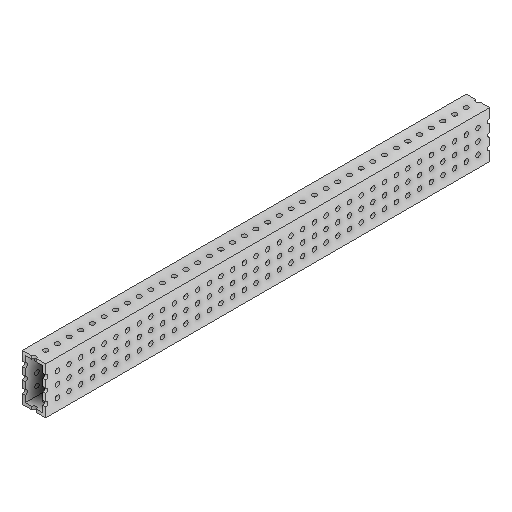
# Autodesk Inventor part: Forja - Base Chassi
Saved by Autodesk Inventor 2027.1 (Build 311270010, 270A)
## iProperties
Created: 2026-05-13
Part Number: Forja - Base Chassi
Material: Genérico
Document SubType Name: Modeling
Designer: djair.oliveira
Density: 1 g/cm^3
Appearance: Padrão
Author: djair.oliveira
Autodesk Inventor part; units mm, degrees
ref_plane "YZ Plane" through (0, 0, 0) normal (1, 0, 0) x (0, 1, 0)
ref_plane "XZ Plane" through (0, 0, 0) normal (0, 1, 0) x (-1, 0, 0)
ref_plane "XY Plane" through (0, 0, 0) normal (0, 0, 1) x (1, 0, 0)
sketch "Esboço1" plane through (0, 0, 0) normal (0, 0, 1) x (1, 0, 0)
  line L0 (12.7, -25.4) -> (-12.7, -25.4)
  line L1 (-12.7, -25.4) -> (-12.7, 25.4)
  line L2 (-12.7, 25.4) -> (12.7, 25.4)
  line L3 (12.7, 25.4) -> (12.7, -25.4)
  line L4 (12.7, -25.4) -> (-12.7, 25.4) construction
  line L5 (-12.7, -25.4) -> (12.7, 25.4) construction
  line L6 (9.525, -22.225) -> (-9.525, -22.225)
  line L7 (-9.525, -22.225) -> (-9.525, 22.225)
  line L8 (-9.525, 22.225) -> (9.525, 22.225)
  line L9 (9.525, 22.225) -> (9.525, -22.225)
  line L10 (9.525, -22.225) -> (-9.525, 22.225) construction
  line L11 (-9.525, -22.225) -> (9.525, 22.225) construction
  point P0 (0, 0)
  dimension "d1" = 3.175
  dimension "d2" = 3.175
  dimension "d3" = 25.4
  dimension "d4" = 50.8
  constraints: 24 end point, 4 midpoint, 4 parallel, 2 horizontal, 2 perpendicular
  measures "d1" distance between parallel lines of L1 L7
  measures "d2" distance between parallel lines of L2 L8
  measures "d3" distance of L1.end L2.end
  measures "d4" distance of L2.end L0.start
extrude "Extrusão1" add sketch "Esboço1" along normal blind 482.6
sketch "Esboço2" plane through (-12.7, 25.4, 0) normal (0, 1, 0) x (1, 0, 0)
  circle A0 centre (12.7, -241.3) radius 2.5
  line L0 (0, 0) -> (0, -482.6) projected
  line L1 (25.4, -482.6) -> (0, -482.6) projected
  line L2 (25.4, 0) -> (0, 0) projected
  circle A1 centre (12.7, -254) radius 2.5
  circle A2 centre (12.7, -228.6) radius 2.5
  circle A3 centre (12.7, -266.7) radius 2.5
  circle A4 centre (12.7, -215.9) radius 2.5
  circle A5 centre (12.7, -279.4) radius 2.5
  circle A6 centre (12.7, -203.2) radius 2.5
  circle A7 centre (12.7, -292.1) radius 2.5
  circle A8 centre (12.7, -190.5) radius 2.5
  circle A9 centre (12.7, -304.8) radius 2.5
  circle A10 centre (12.7, -177.8) radius 2.5
  circle A11 centre (12.7, -317.5) radius 2.5
  circle A12 centre (12.7, -165.1) radius 2.5
  circle A13 centre (12.7, -330.2) radius 2.5
  circle A14 centre (12.7, -152.4) radius 2.5
  circle A15 centre (12.7, -342.9) radius 2.5
  circle A16 centre (12.7, -139.7) radius 2.5
  circle A17 centre (12.7, -355.6) radius 2.5
  circle A18 centre (12.7, -127) radius 2.5
  circle A19 centre (12.7, -368.3) radius 2.5
  circle A20 centre (12.7, -114.3) radius 2.5
  circle A21 centre (12.7, -381) radius 2.5
  circle A22 centre (12.7, -101.6) radius 2.5
  circle A23 centre (12.7, -393.7) radius 2.5
  circle A24 centre (12.7, -88.9) radius 2.5
  circle A25 centre (12.7, -406.4) radius 2.5
  circle A26 centre (12.7, -76.2) radius 2.5
  circle A27 centre (12.7, -419.1) radius 2.5
  circle A28 centre (12.7, -63.5) radius 2.5
  circle A29 centre (12.7, -431.8) radius 2.5
  circle A30 centre (12.7, -50.8) radius 2.5
  circle A31 centre (12.7, -444.5) radius 2.5
  circle A32 centre (12.7, -38.1) radius 2.5
  circle A33 centre (12.7, -457.2) radius 2.5
  circle A34 centre (12.7, -25.4) radius 2.5
  circle A35 centre (12.7, -469.9) radius 2.5
  circle A36 centre (12.7, -12.7) radius 2.5
  circle A37 centre (12.7, -482.6) radius 2.5
  circle A38 centre (12.7, 0) radius 2.5
  circle A39 centre (12.7, -495.3) radius 2.5
  circle A40 centre (12.7, 12.7) radius 2.5
  circle A41 centre (12.7, -508) radius 2.5
  circle A42 centre (12.7, 25.4) radius 2.5
  circle A43 centre (12.7, -520.7) radius 2.5
  circle A44 centre (12.7, 38.1) radius 2.5
  circle A45 centre (12.7, -533.4) radius 2.5
  circle A46 centre (12.7, 50.8) radius 2.5
  circle A47 centre (12.7, -546.1) radius 2.5
  circle A48 centre (12.7, 63.5) radius 2.5
  circle A49 centre (12.7, -558.8) radius 2.5
  circle A50 centre (12.7, 76.2) radius 2.5
  circle A51 centre (12.7, -571.5) radius 2.5
  circle A52 centre (12.7, 88.9) radius 2.5
  circle A53 centre (12.7, -584.2) radius 2.5
  circle A54 centre (12.7, 101.6) radius 2.5
  circle A55 centre (12.7, -596.9) radius 2.5
  circle A56 centre (12.7, 114.3) radius 2.5
  circle A57 centre (12.7, -609.6) radius 2.5
  circle A58 centre (12.7, 127) radius 2.5
  circle A59 centre (12.7, -622.3) radius 2.5
  circle A60 centre (12.7, 139.7) radius 2.5
  circle A61 centre (12.7, -635) radius 2.5
  circle A62 centre (12.7, 152.4) radius 2.5
  circle A63 centre (12.7, -647.7) radius 2.5
  circle A64 centre (12.7, 165.1) radius 2.5
  circle A65 centre (12.7, -660.4) radius 2.5
  circle A66 centre (12.7, 177.8) radius 2.5
  circle A67 centre (12.7, -673.1) radius 2.5
  circle A68 centre (12.7, 190.5) radius 2.5
  circle A69 centre (12.7, -685.8) radius 2.5
  circle A70 centre (12.7, 203.2) radius 2.5
  point P0 (12.7, 0)
  point P1 (12.7, -482.6)
  point P2 (12.7, 0)
  point P3 (12.7, 0)
  dimension "d7" = 5
  dimension "d8" = 12.7
  dimension "d9" = 482.6
  dimension "d10" = 241.3
  dimension "d13" = 12.7
  constraints: 71 centre point, 3 midpoint, 1 vertical, 140 other
  measures "d7" diameter of A0
  measures "d8" distance from line of L0 A0.centre
  measures "d9" distance of point (12.7, -482.6) point (12.7, 0)
  measures "d10" distance of point (12.7, 0) A0.centre
  measures "d13" distance of A0.centre A1.centre
extrude "Extrusão2" cut sketch "Esboço2" against normal up to surface (50.8 mm away)
sketch "Esboço3" plane through (12.7, -25.4, 0) normal (1, 0, 0) x (0, 0, -1)
  circle A0 centre (-241.3, 38.1) radius 2.5
  circle A1 centre (-241.3, 25.4) radius 2.5
  circle A2 centre (-241.3, 12.7) radius 2.5
  line L0 (0, 50.8) -> (-482.6, 50.8) projected
  line L1 (-241.3, 50.8) -> (-241.3, 0)
  line L2 (0, 0) -> (-482.6, 0) projected
  circle A3 centre (-254, 38.1) radius 2.5
  circle A4 centre (-254, 25.4) radius 2.5
  circle A5 centre (-254, 12.7) radius 2.5
  circle A6 centre (-228.6, 38.1) radius 2.5
  circle A7 centre (-228.6, 25.4) radius 2.5
  circle A8 centre (-228.6, 12.7) radius 2.5
  circle A9 centre (-266.7, 38.1) radius 2.5
  circle A10 centre (-266.7, 25.4) radius 2.5
  circle A11 centre (-266.7, 12.7) radius 2.5
  circle A12 centre (-215.9, 38.1) radius 2.5
  circle A13 centre (-215.9, 25.4) radius 2.5
  circle A14 centre (-215.9, 12.7) radius 2.5
  circle A15 centre (-279.4, 38.1) radius 2.5
  circle A16 centre (-279.4, 25.4) radius 2.5
  circle A17 centre (-279.4, 12.7) radius 2.5
  circle A18 centre (-203.2, 38.1) radius 2.5
  circle A19 centre (-203.2, 25.4) radius 2.5
  circle A20 centre (-203.2, 12.7) radius 2.5
  circle A21 centre (-292.1, 38.1) radius 2.5
  circle A22 centre (-292.1, 25.4) radius 2.5
  circle A23 centre (-292.1, 12.7) radius 2.5
  circle A24 centre (-190.5, 38.1) radius 2.5
  circle A25 centre (-190.5, 25.4) radius 2.5
  circle A26 centre (-190.5, 12.7) radius 2.5
  circle A27 centre (-304.8, 38.1) radius 2.5
  circle A28 centre (-304.8, 25.4) radius 2.5
  circle A29 centre (-304.8, 12.7) radius 2.5
  circle A30 centre (-177.8, 38.1) radius 2.5
  circle A31 centre (-177.8, 25.4) radius 2.5
  circle A32 centre (-177.8, 12.7) radius 2.5
  circle A33 centre (-317.5, 38.1) radius 2.5
  circle A34 centre (-317.5, 25.4) radius 2.5
  circle A35 centre (-317.5, 12.7) radius 2.5
  circle A36 centre (-165.1, 38.1) radius 2.5
  circle A37 centre (-165.1, 25.4) radius 2.5
  circle A38 centre (-165.1, 12.7) radius 2.5
  circle A39 centre (-330.2, 38.1) radius 2.5
  circle A40 centre (-330.2, 25.4) radius 2.5
  circle A41 centre (-330.2, 12.7) radius 2.5
  circle A42 centre (-152.4, 38.1) radius 2.5
  circle A43 centre (-152.4, 25.4) radius 2.5
  circle A44 centre (-152.4, 12.7) radius 2.5
  circle A45 centre (-342.9, 38.1) radius 2.5
  circle A46 centre (-342.9, 25.4) radius 2.5
  circle A47 centre (-342.9, 12.7) radius 2.5
  circle A48 centre (-139.7, 38.1) radius 2.5
  circle A49 centre (-139.7, 25.4) radius 2.5
  circle A50 centre (-139.7, 12.7) radius 2.5
  circle A51 centre (-355.6, 38.1) radius 2.5
  circle A52 centre (-355.6, 25.4) radius 2.5
  circle A53 centre (-355.6, 12.7) radius 2.5
  circle A54 centre (-127, 38.1) radius 2.5
  circle A55 centre (-127, 25.4) radius 2.5
  circle A56 centre (-127, 12.7) radius 2.5
  circle A57 centre (-368.3, 38.1) radius 2.5
  circle A58 centre (-368.3, 25.4) radius 2.5
  circle A59 centre (-368.3, 12.7) radius 2.5
  circle A60 centre (-114.3, 38.1) radius 2.5
  circle A61 centre (-114.3, 25.4) radius 2.5
  circle A62 centre (-114.3, 12.7) radius 2.5
  circle A63 centre (-381, 38.1) radius 2.5
  circle A64 centre (-381, 25.4) radius 2.5
  circle A65 centre (-381, 12.7) radius 2.5
  circle A66 centre (-101.6, 38.1) radius 2.5
  circle A67 centre (-101.6, 25.4) radius 2.5
  circle A68 centre (-101.6, 12.7) radius 2.5
  circle A69 centre (-393.7, 38.1) radius 2.5
  circle A70 centre (-393.7, 25.4) radius 2.5
  circle A71 centre (-393.7, 12.7) radius 2.5
  circle A72 centre (-88.9, 38.1) radius 2.5
  circle A73 centre (-88.9, 25.4) radius 2.5
  circle A74 centre (-88.9, 12.7) radius 2.5
  circle A75 centre (-406.4, 38.1) radius 2.5
  circle A76 centre (-406.4, 25.4) radius 2.5
  circle A77 centre (-406.4, 12.7) radius 2.5
  circle A78 centre (-76.2, 38.1) radius 2.5
  circle A79 centre (-76.2, 25.4) radius 2.5
  circle A80 centre (-76.2, 12.7) radius 2.5
  circle A81 centre (-419.1, 38.1) radius 2.5
  circle A82 centre (-419.1, 25.4) radius 2.5
  circle A83 centre (-419.1, 12.7) radius 2.5
  circle A84 centre (-63.5, 38.1) radius 2.5
  circle A85 centre (-63.5, 25.4) radius 2.5
  circle A86 centre (-63.5, 12.7) radius 2.5
  circle A87 centre (-431.8, 38.1) radius 2.5
  circle A88 centre (-431.8, 25.4) radius 2.5
  circle A89 centre (-431.8, 12.7) radius 2.5
  circle A90 centre (-50.8, 38.1) radius 2.5
  circle A91 centre (-50.8, 25.4) radius 2.5
  circle A92 centre (-50.8, 12.7) radius 2.5
  circle A93 centre (-444.5, 38.1) radius 2.5
  circle A94 centre (-444.5, 25.4) radius 2.5
  circle A95 centre (-444.5, 12.7) radius 2.5
  circle A96 centre (-38.1, 38.1) radius 2.5
  circle A97 centre (-38.1, 25.4) radius 2.5
  circle A98 centre (-38.1, 12.7) radius 2.5
  circle A99 centre (-457.2, 38.1) radius 2.5
  circle A100 centre (-457.2, 25.4) radius 2.5
  circle A101 centre (-457.2, 12.7) radius 2.5
  circle A102 centre (-25.4, 38.1) radius 2.5
  circle A103 centre (-25.4, 25.4) radius 2.5
  circle A104 centre (-25.4, 12.7) radius 2.5
  circle A105 centre (-469.9, 38.1) radius 2.5
  circle A106 centre (-469.9, 25.4) radius 2.5
  circle A107 centre (-469.9, 12.7) radius 2.5
  circle A108 centre (-12.7, 38.1) radius 2.5
  circle A109 centre (-12.7, 25.4) radius 2.5
  circle A110 centre (-12.7, 12.7) radius 2.5
  circle A111 centre (-482.6, 38.1) radius 2.5
  circle A112 centre (-482.6, 25.4) radius 2.5
  circle A113 centre (-482.6, 12.7) radius 2.5
  circle A114 centre (0, 38.1) radius 2.5
  circle A115 centre (0, 25.4) radius 2.5
  circle A116 centre (0, 12.7) radius 2.5
  circle A117 centre (-495.3, 38.1) radius 2.5
  circle A118 centre (-495.3, 25.4) radius 2.5
  circle A119 centre (-495.3, 12.7) radius 2.5
  circle A120 centre (12.7, 38.1) radius 2.5
  circle A121 centre (12.7, 25.4) radius 2.5
  circle A122 centre (12.7, 12.7) radius 2.5
  circle A123 centre (-508, 38.1) radius 2.5
  circle A124 centre (-508, 25.4) radius 2.5
  circle A125 centre (-508, 12.7) radius 2.5
  circle A126 centre (25.4, 38.1) radius 2.5
  circle A127 centre (25.4, 25.4) radius 2.5
  circle A128 centre (25.4, 12.7) radius 2.5
  circle A129 centre (-520.7, 38.1) radius 2.5
  circle A130 centre (-520.7, 25.4) radius 2.5
  circle A131 centre (-520.7, 12.7) radius 2.5
  circle A132 centre (38.1, 38.1) radius 2.5
  circle A133 centre (38.1, 25.4) radius 2.5
  circle A134 centre (38.1, 12.7) radius 2.5
  circle A135 centre (-533.4, 38.1) radius 2.5
  circle A136 centre (-533.4, 25.4) radius 2.5
  circle A137 centre (-533.4, 12.7) radius 2.5
  circle A138 centre (50.8, 38.1) radius 2.5
  circle A139 centre (50.8, 25.4) radius 2.5
  circle A140 centre (50.8, 12.7) radius 2.5
  circle A141 centre (-546.1, 38.1) radius 2.5
  circle A142 centre (-546.1, 25.4) radius 2.5
  circle A143 centre (-546.1, 12.7) radius 2.5
  circle A144 centre (63.5, 38.1) radius 2.5
  circle A145 centre (63.5, 25.4) radius 2.5
  circle A146 centre (63.5, 12.7) radius 2.5
  circle A147 centre (-558.8, 38.1) radius 2.5
  circle A148 centre (-558.8, 25.4) radius 2.5
  circle A149 centre (-558.8, 12.7) radius 2.5
  circle A150 centre (76.2, 38.1) radius 2.5
  circle A151 centre (76.2, 25.4) radius 2.5
  circle A152 centre (76.2, 12.7) radius 2.5
  circle A153 centre (-571.5, 38.1) radius 2.5
  circle A154 centre (-571.5, 25.4) radius 2.5
  circle A155 centre (-571.5, 12.7) radius 2.5
  circle A156 centre (88.9, 38.1) radius 2.5
  circle A157 centre (88.9, 25.4) radius 2.5
  circle A158 centre (88.9, 12.7) radius 2.5
  circle A159 centre (-584.2, 38.1) radius 2.5
  circle A160 centre (-584.2, 25.4) radius 2.5
  circle A161 centre (-584.2, 12.7) radius 2.5
  circle A162 centre (101.6, 38.1) radius 2.5
  circle A163 centre (101.6, 25.4) radius 2.5
  circle A164 centre (101.6, 12.7) radius 2.5
  circle A165 centre (-596.9, 38.1) radius 2.5
  circle A166 centre (-596.9, 25.4) radius 2.5
  circle A167 centre (-596.9, 12.7) radius 2.5
  circle A168 centre (114.3, 38.1) radius 2.5
  circle A169 centre (114.3, 25.4) radius 2.5
  circle A170 centre (114.3, 12.7) radius 2.5
  circle A171 centre (-609.6, 38.1) radius 2.5
  circle A172 centre (-609.6, 25.4) radius 2.5
  circle A173 centre (-609.6, 12.7) radius 2.5
  circle A174 centre (127, 38.1) radius 2.5
  circle A175 centre (127, 25.4) radius 2.5
  circle A176 centre (127, 12.7) radius 2.5
  circle A177 centre (-622.3, 38.1) radius 2.5
  circle A178 centre (-622.3, 25.4) radius 2.5
  circle A179 centre (-622.3, 12.7) radius 2.5
  circle A180 centre (139.7, 38.1) radius 2.5
  circle A181 centre (139.7, 25.4) radius 2.5
  circle A182 centre (139.7, 12.7) radius 2.5
  circle A183 centre (-635, 38.1) radius 2.5
  circle A184 centre (-635, 25.4) radius 2.5
  circle A185 centre (-635, 12.7) radius 2.5
  circle A186 centre (152.4, 38.1) radius 2.5
  circle A187 centre (152.4, 25.4) radius 2.5
  circle A188 centre (152.4, 12.7) radius 2.5
  circle A189 centre (-647.7, 38.1) radius 2.5
  circle A190 centre (-647.7, 25.4) radius 2.5
  circle A191 centre (-647.7, 12.7) radius 2.5
  circle A192 centre (165.1, 38.1) radius 2.5
  circle A193 centre (165.1, 25.4) radius 2.5
  circle A194 centre (165.1, 12.7) radius 2.5
  circle A195 centre (-660.4, 38.1) radius 2.5
  circle A196 centre (-660.4, 25.4) radius 2.5
  circle A197 centre (-660.4, 12.7) radius 2.5
  circle A198 centre (177.8, 38.1) radius 2.5
  circle A199 centre (177.8, 25.4) radius 2.5
  circle A200 centre (177.8, 12.7) radius 2.5
  circle A201 centre (-673.1, 38.1) radius 2.5
  circle A202 centre (-673.1, 25.4) radius 2.5
  circle A203 centre (-673.1, 12.7) radius 2.5
  circle A204 centre (190.5, 38.1) radius 2.5
  circle A205 centre (190.5, 25.4) radius 2.5
  circle A206 centre (190.5, 12.7) radius 2.5
  circle A207 centre (-685.8, 38.1) radius 2.5
  circle A208 centre (-685.8, 25.4) radius 2.5
  circle A209 centre (-685.8, 12.7) radius 2.5
  circle A210 centre (203.2, 38.1) radius 2.5
  circle A211 centre (203.2, 25.4) radius 2.5
  circle A212 centre (203.2, 12.7) radius 2.5
  dimension "d20" = 5
  dimension "d21" = 25.4
  dimension "d22" = 12.7
  dimension "d23" = 12.7
  dimension "d26" = 12.7
  constraints: 213 centre point, 2 end point, 2 equal radius, 2 midpoint, 2 vertical alignment, 1 horizontal, 1 point on line, 420 other
  measures "d20" diameter of A1
  measures "d21" distance from line of L0 A1.centre
  measures "d22" distance of A0.centre A1.centre
  measures "d23" distance of A2.centre A1.centre
  measures "d26" distance of A0.centre A3.centre
extrude "Extrusão3" cut sketch "Esboço3" against normal up to surface (25.4 mm away)
equation "\"d2\" = d1"
equation "\"d10\" = 0.5 * d9"
equation "\"d23\" = d22"
